Autodesk Inventor part; units mm, degrees
note: some values were not read from the file. Chosen so that the rebuilt part matches the saved one: direction of "Hole2".
(part 7 of 20)
  line L1382 (-10069.986148, -10024.709041) -> (-10070.005021, -10024.908148)
  line L1383 (-10070.235032, -10024.68545) -> (-10069.986148, -10024.709041)
  line L1384 (-10070.235026, -10024.68555) -> (-10070.235032, -10024.68545)
  line L1385 (-10069.009483, -10025.002511) -> (-10070.005021, -10024.908148)
  line L1386 (-10070.235032, -10024.68545) -> (-10070.055742, -10022.793928)
  line L1387 (-10068.562436, -10022.935473) -> (-10068.741726, -10024.826995)
  line L1388 (-10069.787985, -10022.618411) -> (-10068.792448, -10022.712774)
  line L1389 (-10068.562436, -10022.935473) -> (-10068.81132, -10022.911882)
  line L1390 (-10068.81132, -10022.911882) -> (-10068.792448, -10022.712774)
  line L1391 (-10068.792448, -10022.712774) -> (-10068.792441, -10022.712875)
  line L1392 (-10068.56243, -10022.935573) -> (-10068.562436, -10022.935473)
  line L1393 (-10069.787985, -10022.618411) -> (-10069.806858, -10022.817519)
  line L1394 (-10069.806858, -10022.817519) -> (-10070.055742, -10022.793928)
  line L1395 (-10069.967275, -10024.509933) -> (-10069.825731, -10023.016626)
  line L1396 (-10069.825731, -10023.016626) -> (-10068.830193, -10023.11099)
  line L1397 (-10068.830193, -10023.11099) -> (-10068.971738, -10024.604296)
  line L1398 (-10068.971738, -10024.604296) -> (-10069.967275, -10024.509933)
  line L1399 (-10069.666825, -10023.208877) -> (-10069.775092, -10024.351103)
  line L1400 (-10069.825731, -10023.016626) -> (-10069.666825, -10023.208877)
  line L1401 (-10069.967275, -10024.509933) -> (-10069.775092, -10024.351103)
  line L1402 (-10069.775092, -10024.351103) -> (-10069.130635, -10024.412189)
  line L1403 (-10068.971738, -10024.604296) -> (-10069.130635, -10024.412189)
  line L1404 (-10069.130635, -10024.412189) -> (-10069.022367, -10023.269963)
  line L1405 (-10068.830193, -10023.11099) -> (-10069.022367, -10023.269963)
  line L1406 (-10069.022367, -10023.269963) -> (-10069.666825, -10023.208877)
  circle A29 centre (-10069.423446, -10024.071258) radius 0.1
  line L1407 (-10069.258836, -10023.924227) -> (-10069.289393, -10024.246605)
  line L1408 (-10069.289393, -10024.246605) -> (-10069.588054, -10024.218296)
  line L1409 (-10069.289392, -10024.246619) -> (-10069.588054, -10024.21831)
  line L1410 (-10069.588054, -10024.218296) -> (-10069.557498, -10023.895918)
  line L1411 (-10069.557498, -10023.895918) -> (-10069.258836, -10023.924227)
  line L1412 (-10080.829661, -10022.531991) -> (-10080.630553, -10022.531991)
  line L1413 (-10080.630553, -10022.531991) -> (-10080.630553, -10022.781991)
  line L1414 (-10080.630553, -10021.531991) -> (-10080.829661, -10021.531991)
  line L1415 (-10080.630553, -10021.281991) -> (-10080.630553, -10021.531991)
  line L1416 (-10080.829661, -10022.531991) -> (-10080.829661, -10021.531991)
  line L1417 (-10080.630553, -10021.281991) -> (-10078.824469, -10021.281991)
  line L1418 (-10078.824469, -10022.781991) -> (-10080.630553, -10022.781991)
  line L1419 (-10080.431445, -10021.531991) -> (-10079.023383, -10021.531991)
  line L1420 (-10079.023383, -10022.531991) -> (-10080.431445, -10022.531991)
  line L1421 (-10080.431445, -10022.531991) -> (-10080.431445, -10021.531991)
  line L1422 (-10079.680879, -10021.708318) -> (-10080.161579, -10021.708318)
  line L1423 (-10080.431445, -10021.531991) -> (-10080.161579, -10021.708318)
  line L1424 (-10080.161579, -10021.708318) -> (-10080.161579, -10022.355664)
  line L1425 (-10080.431445, -10022.531991) -> (-10080.161579, -10022.355664)
  line L1426 (-10080.161579, -10022.355664) -> (-10079.680879, -10022.355664)
  ellipse E657 centre (-10079.874789, -10022.031991) end of major axis (-10079.874789, -10021.931991) minor radius 0.099554
  ellipse E658 centre (-10079.870072, -10022.031991) end of major axis (-10079.870072, -10021.931991) minor radius 0.099554 (-10079.870072, -10022.131991) -> (-10079.870072, -10021.931991) ccw
  line L1427 (-10079.870072, -10022.131991) -> (-10079.874789, -10022.131991)
  line L1428 (-10079.870072, -10021.931991) -> (-10079.874789, -10021.931991)
  line L1429 (-10079.708883, -10022.181991) -> (-10080.031262, -10022.181991)
  line L1430 (-10079.690018, -10022.181991) -> (-10079.708883, -10022.181991)
  line L1431 (-10080.031262, -10022.181991) -> (-10080.031262, -10021.881991)
  line L1432 (-10080.031262, -10021.881991) -> (-10079.708883, -10021.881991)
  line L1433 (-10079.690018, -10021.881991) -> (-10079.708883, -10021.881991)
  line L1434 (-10079.708883, -10021.881991) -> (-10079.708883, -10022.181991)
  line L1435 (-10079.690018, -10021.881991) -> (-10079.690018, -10022.181991)
  line L1436 (-10070.252033, -10020.246991) -> (-10070.252033, -10020.046991)
  line L1437 (-10070.221551, -10020.246991) -> (-10070.252033, -10020.246991)
  line L1438 (-10070.003148, -10020.046991) -> (-10069.973178, -10020.046991)
  line L1439 (-10070.252033, -10020.046991) -> (-10070.003148, -10020.046991)
  line L1440 (-10071.247575, -10020.046991) -> (-10071.247575, -10020.246991)
  line L1441 (-10071.49646, -10020.046991) -> (-10071.247575, -10020.046991)
  line L1442 (-10070.252033, -10020.246991) -> (-10071.247575, -10020.246991)
  line L1443 (-10071.49646, -10020.046991) -> (-10071.49646, -10018.146991)
  line L1444 (-10070.003148, -10018.146991) -> (-10070.003148, -10020.046991)
  line L1445 (-10071.247575, -10017.946991) -> (-10070.252033, -10017.946991)
  line L1446 (-10070.003148, -10018.146991) -> (-10070.252033, -10018.146991)
  line L1447 (-10070.252033, -10018.146991) -> (-10070.252033, -10017.946991)
  line L1448 (-10070.252033, -10017.946991) -> (-10070.221551, -10017.946991)
  line L1449 (-10069.973178, -10018.146991) -> (-10070.003148, -10018.146991)
  line L1450 (-10071.247575, -10017.946991) -> (-10071.247575, -10018.146991)
  line L1451 (-10071.247575, -10018.146991) -> (-10071.49646, -10018.146991)
  line L1452 (-10071.247575, -10019.846991) -> (-10071.247575, -10018.346991)
  line L1453 (-10071.247575, -10018.346991) -> (-10070.252033, -10018.346991)
  line L1454 (-10070.252033, -10018.346991) -> (-10070.252033, -10019.846991)
  line L1455 (-10070.252033, -10019.846991) -> (-10071.247575, -10019.846991)
  line L1456 (-10071.247575, -10018.346991) -> (-10071.154859, -10018.40757)
  line L1457 (-10071.247575, -10019.846991) -> (-10071.154859, -10019.786412)
  line L1458 (-10070.252033, -10019.846991) -> (-10070.27838, -10019.78979)
  line L1459 (-10070.252033, -10018.346991) -> (-10070.27838, -10018.404192)
  line L1460 (-10068.792448, -10015.481207) -> (-10068.81132, -10015.2821)
  line L1461 (-10068.792441, -10015.481107) -> (-10068.792448, -10015.481207)
  line L1462 (-10068.562436, -10015.258509) -> (-10068.56243, -10015.258409)
  line L1463 (-10068.81132, -10015.2821) -> (-10068.562436, -10015.258509)
  line L1464 (-10069.806858, -10015.376463) -> (-10069.787985, -10015.57557)
  line L1465 (-10070.055742, -10015.400054) -> (-10069.806858, -10015.376463)
  line L1466 (-10068.792448, -10015.481207) -> (-10069.787985, -10015.57557)
  line L1467 (-10070.055742, -10015.400054) -> (-10070.235032, -10013.508532)
  line L1468 (-10068.741726, -10013.366987) -> (-10068.562436, -10015.258509)
  line L1469 (-10070.005021, -10013.285833) -> (-10069.009483, -10013.19147)
  line L1470 (-10070.235032, -10013.508532) -> (-10070.235026, -10013.508431)
  line L1471 (-10070.005021, -10013.285833) -> (-10069.986148, -10013.484941)
  line L1472 (-10069.986148, -10013.484941) -> (-10070.235032, -10013.508532)
  line L1473 (-10070.005014, -10013.285733) -> (-10070.005021, -10013.285833)
  line L1474 (-10068.741726, -10013.366987) -> (-10068.99061, -10013.390578)
  line L1475 (-10068.99061, -10013.390578) -> (-10069.009483, -10013.19147)
  line L1476 (-10069.009483, -10013.19147) -> (-10069.009477, -10013.19137)
  line L1477 (-10068.99061, -10013.390578) -> (-10068.990604, -10013.390478)
  line L1478 (-10068.74172, -10013.366887) -> (-10068.741726, -10013.366987)
  line L1479 (-10069.825731, -10015.177355) -> (-10069.967275, -10013.684048)
  line L1480 (-10069.967275, -10013.684048) -> (-10068.971738, -10013.589685)
  line L1481 (-10068.971738, -10013.589685) -> (-10068.830193, -10015.082992)
  line L1482 (-10068.830193, -10015.082992) -> (-10069.825731, -10015.177355)
  line L1483 (-10069.775092, -10013.842878) -> (-10069.666825, -10014.985105)
  line L1484 (-10069.967275, -10013.684048) -> (-10069.775092, -10013.842878)
  line L1485 (-10069.825731, -10015.177355) -> (-10069.666825, -10014.985105)
  line L1486 (-10069.666825, -10014.985105) -> (-10069.022367, -10014.924019)
  line L1487 (-10068.830193, -10015.082992) -> (-10069.022367, -10014.924019)
  line L1488 (-10069.022367, -10014.924019) -> (-10069.130635, -10013.781793)
  line L1489 (-10068.971738, -10013.589685) -> (-10069.130635, -10013.781793)
  line L1490 (-10069.130635, -10013.781793) -> (-10069.775092, -10013.842878)
  circle A30 centre (-10069.374016, -10014.644209) radius 0.1
  line L1491 (-10069.239964, -10014.468862) -> (-10069.209407, -10014.79124)
  line L1492 (-10069.209407, -10014.79124) -> (-10069.508068, -10014.819549)
  line L1493 (-10069.508068, -10014.819549) -> (-10069.538625, -10014.497171)
  line L1494 (-10069.538625, -10014.497171) -> (-10069.239964, -10014.468862)
  line L1495 (-10069.538624, -10014.497157) -> (-10069.239963, -10014.468848)
  line L1496 (-10051.002001, -10021.596991) -> (-10051.202001, -10021.596991)
  line L1497 (-10051.202001, -10021.596991) -> (-10051.202001, -10021.346991)
  line L1498 (-10051.202001, -10022.596991) -> (-10051.002001, -10022.596991)
  line L1499 (-10051.202001, -10022.846991) -> (-10051.202001, -10022.596991)
  line L1500 (-10051.002001, -10021.596991) -> (-10051.002001, -10022.596991)
  line L1501 (-10051.202001, -10022.846991) -> (-10053.102001, -10022.846991)
  line L1502 (-10053.102001, -10021.346991) -> (-10051.202001, -10021.346991)
  line L1503 (-10053.302001, -10022.596991) -> (-10053.302001, -10021.596991)
  line L1504 (-10053.102001, -10021.346991) -> (-10053.102001, -10021.596991)
  line L1505 (-10053.102001, -10021.596991) -> (-10053.302001, -10021.596991)
  line L1506 (-10053.302001, -10022.596991) -> (-10053.102001, -10022.596991)
  line L1507 (-10053.102001, -10022.596991) -> (-10053.102001, -10022.846991)
  line L1508 (-10051.402001, -10022.596991) -> (-10052.902001, -10022.596991)
  line L1509 (-10052.902001, -10022.596991) -> (-10052.902001, -10021.596991)
  line L1510 (-10052.902001, -10021.596991) -> (-10051.402001, -10021.596991)
  line L1511 (-10051.402001, -10021.596991) -> (-10051.402001, -10022.596991)
  line L1512 (-10052.725674, -10022.420664) -> (-10051.578328, -10022.420664)
  line L1513 (-10052.902001, -10022.596991) -> (-10052.725674, -10022.420664)
  line L1514 (-10051.402001, -10022.596991) -> (-10051.578328, -10022.420664)
  line L1515 (-10051.578328, -10022.420664) -> (-10051.578328, -10021.773318)
  line L1516 (-10051.402001, -10021.596991) -> (-10051.578328, -10021.773318)
  line L1517 (-10051.578328, -10021.773318) -> (-10052.725674, -10021.773318)
  line L1518 (-10052.902001, -10021.596991) -> (-10052.725674, -10021.773318)
  line L1519 (-10052.725674, -10021.773318) -> (-10052.725674, -10022.420664)
  circle A31 centre (-10051.890089, -10022.096991) radius 0.1
  line L1520 (-10052.052001, -10021.946991) -> (-10051.728178, -10021.946991)
  line L1521 (-10051.728178, -10021.946991) -> (-10051.728178, -10022.246991)
  line L1522 (-10051.728178, -10022.246991) -> (-10052.052001, -10022.246991)
  line L1523 (-10052.052001, -10022.246991) -> (-10052.052001, -10021.946991)
  line L1524 (-10061.600001, -10017.946991) -> (-10061.600001, -10018.146991)
  line L1525 (-10061.600001, -10018.146991) -> (-10061.850001, -10018.146991)
  line L1526 (-10060.600001, -10018.146991) -> (-10060.600001, -10017.946991)
  line L1527 (-10060.350001, -10018.146991) -> (-10060.600001, -10018.146991)
  line L1528 (-10061.600001, -10017.946991) -> (-10060.600001, -10017.946991)
  line L1529 (-10060.350001, -10018.146991) -> (-10060.350001, -10020.046991)
  line L1530 (-10061.850001, -10020.046991) -> (-10061.850001, -10018.146991)
  line L1531 (-10060.600001, -10020.246991) -> (-10061.600001, -10020.246991)
  line L1532 (-10061.850001, -10020.046991) -> (-10061.600001, -10020.046991)
  line L1533 (-10061.600001, -10020.046991) -> (-10061.600001, -10020.246991)
  line L1534 (-10060.600001, -10020.246991) -> (-10060.600001, -10020.046991)
  line L1535 (-10060.600001, -10020.046991) -> (-10060.350001, -10020.046991)
  line L1536 (-10060.600001, -10018.346991) -> (-10060.600001, -10019.846991)
  line L1537 (-10060.600001, -10019.846991) -> (-10061.600001, -10019.846991)
  line L1538 (-10061.600001, -10019.846991) -> (-10061.600001, -10018.346991)
  line L1539 (-10061.600001, -10018.346991) -> (-10060.600001, -10018.346991)
  line L1540 (-10060.776328, -10019.670664) -> (-10060.776328, -10018.523318)
  line L1541 (-10060.600001, -10019.846991) -> (-10060.776328, -10019.670664)
  line L1542 (-10060.600001, -10018.346991) -> (-10060.776328, -10018.523318)
  line L1543 (-10060.776328, -10018.523318) -> (-10061.423674, -10018.523318)
  line L1544 (-10061.600001, -10018.346991) -> (-10061.423674, -10018.523318)
  line L1545 (-10061.423674, -10018.523318) -> (-10061.423674, -10019.670664)
  line L1546 (-10061.600001, -10019.846991) -> (-10061.423674, -10019.670664)
  line L1547 (-10061.423674, -10019.670664) -> (-10060.776328, -10019.670664)
  circle A32 centre (-10061.100001, -10018.835079) radius 0.1
  line L1548 (-10061.250001, -10018.996991) -> (-10061.250001, -10018.673168)
  line L1549 (-10061.250001, -10018.673168) -> (-10060.950001, -10018.673168)
  line L1550 (-10060.950001, -10018.673168) -> (-10060.950001, -10018.996991)
  line L1551 (-10060.950001, -10018.996991) -> (-10061.250001, -10018.996991)
  line L1552 (-10051.002001, -10015.596991) -> (-10051.202001, -10015.596991)
  line L1553 (-10051.202001, -10015.596991) -> (-10051.202001, -10015.346991)
  line L1554 (-10051.202001, -10016.596991) -> (-10051.002001, -10016.596991)
  line L1555 (-10051.202001, -10016.846991) -> (-10051.202001, -10016.596991)
  line L1556 (-10051.002001, -10015.596991) -> (-10051.002001, -10016.596991)
  line L1557 (-10051.202001, -10016.846991) -> (-10053.102001, -10016.846991)
  line L1558 (-10053.102001, -10015.346991) -> (-10051.202001, -10015.346991)
  line L1559 (-10053.302001, -10016.596991) -> (-10053.302001, -10015.596991)
  line L1560 (-10053.102001, -10015.346991) -> (-10053.102001, -10015.596991)
  line L1561 (-10053.102001, -10015.596991) -> (-10053.302001, -10015.596991)
  line L1562 (-10053.302001, -10016.596991) -> (-10053.102001, -10016.596991)
  line L1563 (-10053.102001, -10016.596991) -> (-10053.102001, -10016.846991)
  line L1564 (-10051.402001, -10016.596991) -> (-10052.902001, -10016.596991)
  line L1565 (-10052.902001, -10016.596991) -> (-10052.902001, -10015.596991)
  line L1566 (-10052.902001, -10015.596991) -> (-10051.402001, -10015.596991)
  line L1567 (-10051.402001, -10015.596991) -> (-10051.402001, -10016.596991)
  line L1568 (-10052.725674, -10016.420664) -> (-10051.578328, -10016.420664)
  line L1569 (-10052.902001, -10016.596991) -> (-10052.725674, -10016.420664)
  line L1570 (-10051.402001, -10016.596991) -> (-10051.578328, -10016.420664)
  line L1571 (-10051.578328, -10016.420664) -> (-10051.578328, -10015.773318)
  line L1572 (-10051.402001, -10015.596991) -> (-10051.578328, -10015.773318)
  line L1573 (-10051.578328, -10015.773318) -> (-10052.725674, -10015.773318)
  line L1574 (-10052.902001, -10015.596991) -> (-10052.725674, -10015.773318)
  line L1575 (-10052.725674, -10015.773318) -> (-10052.725674, -10016.420664)
  circle A33 centre (-10051.890089, -10016.096991) radius 0.1
  line L1576 (-10052.052001, -10015.946991) -> (-10051.728178, -10015.946991)
  line L1577 (-10051.728178, -10015.946991) -> (-10051.728178, -10016.246991)
  line L1578 (-10051.728178, -10016.246991) -> (-10052.052001, -10016.246991)
  line L1579 (-10052.052001, -10016.246991) -> (-10052.052001, -10015.946991)
  line L1580 (-10079.023383, -10015.661991) -> (-10078.824469, -10015.661991)
  line L1581 (-10078.824469, -10015.661991) -> (-10078.824469, -10015.411991)
  line L1582 (-10078.824469, -10016.661991) -> (-10079.023383, -10016.661991)
  line L1583 (-10078.824469, -10016.911991) -> (-10078.824469, -10016.661991)
  line L1584 (-10079.023383, -10015.661991) -> (-10079.023383, -10016.661991)
  line L1585 (-10078.824469, -10016.911991) -> (-10077.066524, -10016.911991)
  line L1586 (-10077.066524, -10015.411991) -> (-10078.824469, -10015.411991)
  line L1587 (-10078.625555, -10016.661991) -> (-10077.265175, -10016.661991)
  line L1588 (-10078.625555, -10015.661991) -> (-10078.625555, -10016.661991)
  line L1589 (-10077.265175, -10015.661991) -> (-10078.625555, -10015.661991)
  line L1590 (-10078.625555, -10016.661991) -> (-10078.372051, -10016.50203)
  line L1591 (-10078.625555, -10015.661991) -> (-10078.372051, -10015.821952)
  ellipse E659 centre (-10078.062063, -10016.161991) end of major axis (-10078.062063, -10016.261991) minor radius 0.099457
  ellipse E660 centre (-10078.056859, -10016.161991) end of major axis (-10078.056859, -10016.261991) minor radius 0.099457 (-10078.056859, -10016.261991) -> (-10078.056859, -10016.061991) ccw
  line L1592 (-10078.062063, -10016.061991) -> (-10078.056859, -10016.061991)
  line L1593 (-10078.062063, -10016.261991) -> (-10078.056859, -10016.261991)
  line L1594 (-10077.895827, -10016.011991) -> (-10078.217892, -10016.011991)
  line L1595 (-10077.88528, -10016.011991) -> (-10077.895827, -10016.011991)
  line L1596 (-10078.217892, -10016.011991) -> (-10078.217892, -10016.311991)
  line L1597 (-10078.217892, -10016.311991) -> (-10077.895827, -10016.311991)
  line L1598 (-10077.88528, -10016.311991) -> (-10077.895827, -10016.311991)
  line L1599 (-10077.895827, -10016.311991) -> (-10077.895827, -10016.011991)
  line L1600 (-10077.691531, -10011.315342) -> (-10077.890346, -10011.336143)
  line L1601 (-10077.890346, -10011.336143) -> (-10077.890422, -10011.336371)
  line L1602 (-10077.890422, -10011.336371) -> (-10077.691508, -10011.31556)
  line L1603 (-10077.691508, -10011.31556) -> (-10077.717522, -10011.066917)
  line L1604 (-10077.717522, -10011.066917) -> (-10077.717446, -10011.066689)
  line L1605 (-10077.58745, -10012.310131) -> (-10077.786364, -10012.330942)
  line L1606 (-10077.561436, -10012.558774) -> (-10077.58745, -10012.310131)
  line L1607 (-10075.973217, -10010.884197) -> (-10077.717446, -10011.066689)
  line L1608 (-10075.498774, -10012.091381) -> (-10075.526412, -10011.827228)
  line L1609 (-10077.890422, -10011.336371) -> (-10077.786364, -10012.330942)
  line L1610 (-10077.561436, -10012.558774) -> (-10075.67175, -10012.361064)
  line L1611 (-10075.49885, -10012.09161) -> (-10075.602908, -10011.097038)
  line L1612 (-10075.827837, -10010.869207) -> (-10077.717522, -10011.066917)
  line L1613 (-10075.671674, -10012.360836) -> (-10075.697666, -10012.112411)
  line L1614 (-10075.67175, -10012.361064) -> (-10075.671674, -10012.360836)
  line L1615 (-10075.697765, -10012.112421) -> (-10075.67175, -10012.361064)
  line L1616 (-10075.49885, -10012.09161) -> (-10075.697765, -10012.112421)
  line L1617 (-10075.498774, -10012.091381) -> (-10075.49885, -10012.09161)
  line L1618 (-10075.801822, -10011.11785) -> (-10075.602908, -10011.097038)
  line L1619 (-10075.827837, -10010.869207) -> (-10075.801822, -10011.11785)
  line L1620 (-10077.388536, -10012.289319) -> (-10075.896679, -10012.133233)
  line L1621 (-10077.492594, -10011.294748) -> (-10077.388536, -10012.289319)
  line L1622 (-10076.000737, -10011.138661) -> (-10077.492594, -10011.294748)
  line L1623 (-10075.896679, -10012.133233) -> (-10076.000737, -10011.138661)
  line L1624 (-10076.090343, -10011.976048) -> (-10077.23146, -10012.095439)
  line L1625 (-10077.388536, -10012.289319) -> (-10077.23146, -10012.095439)
  line L1626 (-10075.896679, -10012.133233) -> (-10076.090343, -10011.976048)
  line L1627 (-10077.23146, -10012.095439) -> (-10077.298821, -10011.451607)
  line L1628 (-10077.492594, -10011.294748) -> (-10077.298821, -10011.451607)
  line L1629 (-10077.298821, -10011.451607) -> (-10076.157704, -10011.332216)
  line L1630 (-10076.000737, -10011.138661) -> (-10076.157704, -10011.332216)
  line L1631 (-10076.157704, -10011.332216) -> (-10076.090343, -10011.976048)
  circle A34 centre (-10076.955085, -10011.741122) radius 0.1
  line L1632 (-10076.809659, -10011.57508) -> (-10077.131723, -10011.608776)
  line L1633 (-10076.809648, -10011.575048) -> (-10076.809659, -10011.57508)
  line L1634 (-10076.809648, -10011.575048) -> (-10077.131713, -10011.608744)
  line L1635 (-10077.131713, -10011.608744) -> (-10077.131723, -10011.608776)
  line L1636 (-10077.131723, -10011.608776) -> (-10077.100506, -10011.907148)
  line L1637 (-10077.100506, -10011.907148) -> (-10076.778441, -10011.873452)
  line L1638 (-10076.77843, -10011.873419) -> (-10076.778441, -10011.873452)
  line L1639 (-10076.778441, -10011.873452) -> (-10076.809659, -10011.57508)
  line L1640 (-10076.77843, -10011.873419) -> (-10076.809648, -10011.575048)
  line L1641 (-10077.265175, -10015.661991) -> (-10077.066524, -10015.661991)
  line L1642 (-10077.066524, -10015.661991) -> (-10077.066524, -10015.411991)
  line L1643 (-10077.066524, -10016.661991) -> (-10077.265175, -10016.661991)
  line L1644 (-10077.066524, -10016.911991) -> (-10077.066524, -10016.661991)
  line L1645 (-10075.017046, -10015.661991) -> (-10075.017046, -10015.411991)
  line L1646 (-10075.179332, -10015.661991) -> (-10074.98068, -10015.661991)
  line L1647 (-10075.179332, -10015.411991) -> (-10075.179332, -10015.661991)
  line L1648 (-10074.98068, -10015.661991) -> (-10074.818395, -10015.661991)
  line L1649 (-10075.017046, -10015.411991) -> (-10075.179332, -10015.411991)
  line L1650 (-10074.818395, -10016.661991) -> (-10074.818395, -10015.661991)
  line L1651 (-10077.265175, -10015.661991) -> (-10077.265175, -10016.661991)
  line L1652 (-10077.066524, -10016.911991) -> (-10075.179332, -10016.911991)
  line L1653 (-10074.98068, -10016.661991) -> (-10074.98068, -10015.661991)
  line L1654 (-10075.179332, -10015.411991) -> (-10077.066524, -10015.411991)
  line L1655 (-10075.017046, -10016.911991) -> (-10075.017046, -10016.661991)
  line L1656 (-10075.179332, -10016.911991) -> (-10075.017046, -10016.911991)
  line L1657 (-10075.179332, -10016.661991) -> (-10075.179332, -10016.911991)
  line L1658 (-10074.98068, -10016.661991) -> (-10075.179332, -10016.661991)
  line L1659 (-10074.818395, -10016.661991) -> (-10074.98068, -10016.661991)
  line L1660 (-10076.867872, -10016.661991) -> (-10075.377984, -10016.661991)
  line L1661 (-10076.867872, -10015.661991) -> (-10076.867872, -10016.661991)
  line L1662 (-10075.377984, -10015.661991) -> (-10076.867872, -10015.661991)
  line L1663 (-10075.377984, -10016.661991) -> (-10075.377984, -10015.661991)
  line L1664 (-10075.437204, -10016.485664) -> (-10076.576815, -10016.485664)
  line L1665 (-10076.867872, -10016.661991) -> (-10076.576815, -10016.485664)
  line L1666 (-10075.377984, -10016.661991) -> (-10075.437204, -10016.485664)
  line L1667 (-10076.576815, -10016.485664) -> (-10076.576815, -10015.838318)
  line L1668 (-10076.867872, -10015.661991) -> (-10076.576815, -10015.838318)
  line L1669 (-10076.576815, -10015.838318) -> (-10075.437204, -10015.838318)
  line L1670 (-10075.377984, -10015.661991) -> (-10075.437204, -10015.838318)
  line L1671 (-10075.437204, -10015.838318) -> (-10075.437204, -10016.485664)
  ellipse E661 centre (-10076.296135, -10016.161991) end of major axis (-10076.296135, -10016.261991) minor radius 0.099326
  ellipse E662 centre (-10076.290339, -10016.161991) end of major axis (-10076.290339, -10016.261991) minor radius 0.099326 (-10076.290339, -10016.261991) -> (-10076.290339, -10016.061991) ccw
  line L1672 (-10076.296135, -10016.061991) -> (-10076.290339, -10016.061991)
  line L1673 (-10076.296135, -10016.261991) -> (-10076.290339, -10016.261991)
  line L1674 (-10076.129519, -10016.011991) -> (-10076.451159, -10016.011991)
  line L1675 (-10076.106335, -10016.011991) -> (-10076.129519, -10016.011991)
  line L1676 (-10076.451159, -10016.011991) -> (-10076.451159, -10016.311991)
  line L1677 (-10076.451159, -10016.311991) -> (-10076.129519, -10016.311991)
  line L1678 (-10076.106335, -10016.311991) -> (-10076.129519, -10016.311991)
  line L1679 (-10076.129519, -10016.311991) -> (-10076.129519, -10016.011991)
  line L1680 (-10076.106335, -10016.311991) -> (-10076.106335, -10016.011991)
  line L1681 (-10076.003508, -10010.624332) -> (-10076.003562, -10010.624474)
  line L1682 (-10076.003562, -10010.624474) -> (-10075.804914, -10010.601264)
  line L1683 (-10075.804914, -10010.601264) -> (-10075.833925, -10010.352953)
  line L1684 (-10075.833925, -10010.352953) -> (-10075.833871, -10010.352812)
  line L1685 (-10073.946708, -10010.132322) -> (-10075.833871, -10010.352812)
  line L1686 (-10073.715814, -10010.385094) -> (-10073.719047, -10010.357424)
  line L1687 (-10076.003562, -10010.624474) -> (-10075.973192, -10010.884415)
  line L1688 (-10075.52651, -10011.827239) -> (-10073.772692, -10011.622329)
  line L1689 (-10073.603055, -10011.350809) -> (-10073.719102, -10010.357565)
  line L1690 (-10073.946762, -10010.132464) -> (-10075.833925, -10010.352953)
  line L1691 (-10073.920953, -10010.352758) -> (-10073.946708, -10010.132322)
  line L1692 (-10073.719047, -10010.357424) -> (-10073.815719, -10010.368718)
  line L1693 (-10073.917751, -10010.380775) -> (-10073.719102, -10010.357565)
  line L1694 (-10073.946762, -10010.132464) -> (-10073.917751, -10010.380775)
  line L1695 (-10073.917751, -10010.380775) -> (-10073.917696, -10010.380633)
  line L1696 (-10073.719102, -10010.357565) -> (-10073.719047, -10010.357424)
  line L1697 (-10073.946708, -10010.132322) -> (-10073.946762, -10010.132464)
  line L1698 (-10073.772692, -10011.622329) -> (-10073.772637, -10011.622188)
  line L1699 (-10073.801703, -10011.374018) -> (-10073.772692, -10011.622329)
  line L1700 (-10073.603055, -10011.350809) -> (-10073.801703, -10011.374018)
  line L1701 (-10073.603, -10011.350667) -> (-10073.603055, -10011.350809)
  line L1702 (-10075.490218, -10011.571299) -> (-10074.000352, -10011.397228)
  line L1703 (-10075.606265, -10010.578055) -> (-10075.490218, -10011.571299)
  line L1704 (-10074.116399, -10010.403984) -> (-10075.606265, -10010.578055)
  line L1705 (-10074.000352, -10011.397228) -> (-10074.116399, -10010.403984)
  line L1706 (-10074.195911, -10011.242453) -> (-10075.335505, -10011.375599)
  line L1707 (-10075.490218, -10011.571299) -> (-10075.335505, -10011.375599)
  line L1708 (-10074.000352, -10011.397228) -> (-10074.195911, -10011.242453)
  line L1709 (-10075.335505, -10011.375599) -> (-10075.410628, -10010.732627)
  line L1710 (-10075.606265, -10010.578055) -> (-10075.410628, -10010.732627)
  line L1711 (-10075.410628, -10010.732627) -> (-10074.271034, -10010.599481)
  line L1712 (-10074.116399, -10010.403984) -> (-10074.271034, -10010.599481)
  line L1713 (-10074.271034, -10010.599481) -> (-10074.195911, -10011.242453)
  circle A35 centre (-10075.063421, -10011.017959) radius 0.1
  line L1714 (-10074.920009, -10010.850179) -> (-10075.241644, -10010.887757)
  line L1715 (-10074.920001, -10010.850158) -> (-10074.920009, -10010.850179)
  line L1716 (-10074.920001, -10010.850158) -> (-10075.241636, -10010.887737)
  line L1717 (-10075.241636, -10010.887737) -> (-10075.241644, -10010.887757)
  line L1718 (-10075.241644, -10010.887757) -> (-10075.20683, -10011.18573)
  line L1719 (-10075.20683, -10011.18573) -> (-10074.885195, -10011.148152)
  line L1720 (-10074.885187, -10011.148131) -> (-10074.885195, -10011.148152)
  line L1721 (-10074.885195, -10011.148152) -> (-10074.920009, -10010.850179)
  line L1722 (-10074.885187, -10011.148131) -> (-10074.920001, -10010.850158)
  line L1723 (-10080.829661, -10015.661991) -> (-10080.630553, -10015.661991)
  line L1724 (-10080.630553, -10015.661991) -> (-10080.630553, -10015.411991)
  line L1725 (-10080.630553, -10016.661991) -> (-10080.829661, -10016.661991)
  line L1726 (-10080.630553, -10016.911991) -> (-10080.630553, -10016.661991)
  line L1727 (-10080.829661, -10015.661991) -> (-10080.829661, -10016.661991)
  line L1728 (-10080.630553, -10016.911991) -> (-10078.824469, -10016.911991)
  line L1729 (-10078.824469, -10015.411991) -> (-10080.630553, -10015.411991)
  line L1730 (-10080.431445, -10016.661991) -> (-10079.023383, -10016.661991)
  line L1731 (-10080.431445, -10015.661991) -> (-10080.431445, -10016.661991)
  line L1732 (-10079.023383, -10015.661991) -> (-10080.431445, -10015.661991)
  line L1733 (-10079.680879, -10016.485664) -> (-10080.161579, -10016.485664)
  line L1734 (-10080.431445, -10016.661991) -> (-10080.161579, -10016.485664)
  line L1735 (-10080.161579, -10016.485664) -> (-10080.161579, -10015.838318)
  line L1736 (-10080.431445, -10015.661991) -> (-10080.161579, -10015.838318)
  line L1737 (-10080.161579, -10015.838318) -> (-10079.680879, -10015.838318)
  ellipse E663 centre (-10079.874789, -10016.161991) end of major axis (-10079.874789, -10016.261991) minor radius 0.099554
  ellipse E664 centre (-10079.870072, -10016.161991) end of major axis (-10079.870072, -10016.261991) minor radius 0.099554 (-10079.870072, -10016.261991) -> (-10079.870072, -10016.061991) ccw
  line L1738 (-10079.874789, -10016.061991) -> (-10079.870072, -10016.061991)
  line L1739 (-10079.874789, -10016.261991) -> (-10079.870072, -10016.261991)
  line L1740 (-10079.708883, -10016.011991) -> (-10080.031262, -10016.011991)
  line L1741 (-10079.690018, -10016.011991) -> (-10079.708883, -10016.011991)
  line L1742 (-10080.031262, -10016.011991) -> (-10080.031262, -10016.311991)
  line L1743 (-10080.031262, -10016.311991) -> (-10079.708883, -10016.311991)
  line L1744 (-10079.690018, -10016.311991) -> (-10079.708883, -10016.311991)
  line L1745 (-10079.708883, -10016.311991) -> (-10079.708883, -10016.011991)
  line L1746 (-10079.690018, -10016.311991) -> (-10079.690018, -10016.011991)
  line L1747 (-10079.603594, -10011.900303) -> (-10079.802686, -10011.919175)
  line L1748 (-10079.802686, -10011.919175) -> (-10079.802692, -10011.919275)
  line L1749 (-10079.802692, -10011.919275) -> (-10079.603585, -10011.900402)
  line L1750 (-10079.603585, -10011.900402) -> (-10079.627175, -10011.651518)
  line L1751 (-10079.627175, -10011.651518) -> (-10079.627169, -10011.651417)
  line L1752 (-10079.509221, -10012.89594) -> (-10079.708329, -10012.914813)
  line L1753 (-10079.485631, -10013.144825) -> (-10079.509221, -10012.89594)
  line L1754 (-10079.407047, -10011.630553) -> (-10079.627169, -10011.651417)
  line L1755 (-10079.802692, -10011.919275) -> (-10079.708329, -10012.914813)
  line L1756 (-10079.485631, -10013.144825) -> (-10077.594109, -10012.965534)
  line L1757 (-10077.418592, -10012.697777) -> (-10077.433041, -10012.54534)
  line L1758 (-10077.874828, -10011.48542) -> (-10079.627175, -10011.651518)
  line L1759 (-10077.594109, -10012.965534) -> (-10077.594103, -10012.965434)
  line L1760 (-10077.6177, -10012.71665) -> (-10077.594109, -10012.965534)
  line L1761 (-10077.418592, -10012.697777) -> (-10077.6177, -10012.71665)
  line L1762 (-10077.418586, -10012.697677) -> (-10077.418592, -10012.697777)
  line L1763 (-10079.310114, -10012.877067) -> (-10077.816807, -10012.735523)
  line L1764 (-10079.404477, -10011.88153) -> (-10079.310114, -10012.877067)
  line L1765 (-10077.91117, -10011.739985) -> (-10079.404477, -10011.88153)
  line L1766 (-10077.816807, -10012.735523) -> (-10077.91117, -10011.739985)
  line L1767 (-10078.008982, -10012.57655) -> (-10079.151208, -10012.684817)
  line L1768 (-10079.310114, -10012.877067) -> (-10079.151208, -10012.684817)
  line L1769 (-10077.816807, -10012.735523) -> (-10078.008982, -10012.57655)
  line L1770 (-10079.151208, -10012.684817) -> (-10079.212294, -10012.040359)
  line L1771 (-10079.404477, -10011.88153) -> (-10079.212294, -10012.040359)
  line L1772 (-10079.212294, -10012.040359) -> (-10078.070067, -10011.932092)
  line L1773 (-10077.91117, -10011.739985) -> (-10078.070067, -10011.932092)
  line L1774 (-10078.070067, -10011.932092) -> (-10078.008982, -10012.57655)
  circle A36 centre (-10078.871381, -10012.333187) radius 0.1
  line L1775 (-10078.724347, -10012.168574) -> (-10079.046725, -10012.199131)
  line L1776 (-10078.724346, -10012.16856) -> (-10079.046724, -10012.199117)
  line L1777 (-10079.046725, -10012.199131) -> (-10079.018416, -10012.497793)
  line L1778 (-10079.018416, -10012.497793) -> (-10078.696038, -10012.467236)
  line L1779 (-10078.696038, -10012.467236) -> (-10078.724347, -10012.168574)
  ellipse E665 centre (-10075.730106, -10029.62245) end of major axis (-10075.669515, -10030.82092) minor radius 0.214474 (-10075.933672, -10028.865824) -> (-10075.631613, -10030.799013) ccw
  ellipse E666 centre (-10075.533577, -10029.612514) end of major axis (-10075.483085, -10030.611239) minor radius 0.178729 (-10075.711061, -10029.080492) -> (-10075.384751, -10030.398789) ccw
  line L1780 (-10075.4515, -10030.592983) -> (-10075.631613, -10030.799013)
  ellipse E667 centre (-10075.533577, -10029.612514) end of major axis (-10075.495708, -10030.361558) minor radius 0.134046 (-10075.671866, -10029.337058) -> (-10075.41406, -10030.151964) ccw
  line L1781 (-10075.669515, -10030.82092) -> (-10076.518016, -10030.863817)
  ellipse E668 centre (-10075.730106, -10008.571531) end of major axis (-10075.669515, -10007.373062) minor radius 0.214474 (-10075.631613, -10007.394969) -> (-10075.933672, -10009.328157) ccw
  ellipse E669 centre (-10075.533577, -10008.581467) end of major axis (-10075.483085, -10007.582743) minor radius 0.178729 (-10075.384751, -10007.795193) -> (-10075.711061, -10009.11349) ccw
  line L1782 (-10075.4515, -10007.600998) -> (-10075.631613, -10007.394969)
  ellipse E670 centre (-10075.533577, -10008.581467) end of major axis (-10075.495708, -10007.832424) minor radius 0.134046 (-10075.41406, -10008.042018) -> (-10075.671866, -10008.856924) ccw
  line L1783 (-10075.669515, -10007.373062) -> (-10076.518016, -10007.330164)
  ellipse E671 centre (-10090.417065, -10019.096991) end of major axis (-10090.417065, -10019.663411) minor radius 0.563895 (-10089.989225, -10018.728017) -> (-10089.989225, -10019.465964) ccw
  line L1784 (-10090.80989, -10019.210594) -> (-10090.711422, -10018.812073)
  line L1785 (-10090.711422, -10018.812073) -> (-10090.318598, -10018.69847)
  line L1786 (-10090.318598, -10018.69847) -> (-10090.048204, -10018.960194)
  line L1787 (-10090.080668, -10019.211762) -> (-10090.122709, -10019.381909)
  line L1788 (-10090.122709, -10019.381909) -> (-10090.515533, -10019.495512)
  line L1789 (-10090.515533, -10019.495512) -> (-10090.80989, -10019.210594)
  line L1790 (-10090.711422, -10018.812073) -> (-10090.621727, -10018.812073)
  line L1791 (-10090.720635, -10019.210594) -> (-10090.80989, -10019.210594)
  spline S53 degree 3 poles (-10045.596901, -10030.692025) (-10045.596275, -10030.687279) (-10045.594915, -10030.676953) (-10045.585272, -10030.662297) (-10045.570743, -10030.647725) (-10045.550423, -10030.633362) (-10045.524771, -10030.619481) (-10045.482006, -10030.600847) (-10045.432986, -10030.585045) (-10045.378486, -10030.571429) (-10045.314115, -10030.55807) (-10045.225805, -10030.544735) (-10045.114584, -10030.535371) (-10045.000001, -10030.532033) (-10044.885417, -10030.535371) (-10044.774196, -10030.544735) (-10044.685886, -10030.55807) (-10044.621515, -10030.571429) (-10044.567015, -10030.585045) (-10044.517995, -10030.600847) (-10044.475231, -10030.619481) (-10044.449578, -10030.633362) (-10044.429258, -10030.647725) (-10044.41473, -10030.662297) (-10044.405087, -10030.676953) (-10044.403726, -10030.687279) (-10044.403101, -10030.692025) knots 0 0 0 0 0.01106677 0.02407754 0.03992786 0.05913986 0.0819337 0.10802006 0.16805875 0.20201508 0.23929564 0.3216678 0.41056278 0.5 0.58943722 0.6783322 0.76070436 0.79798492 0.83194125 0.89197994 0.9180663 0.94086014 0.96007214 0.97592246 0.98893323 1 1 1 1
  spline S54 degree 3 poles (-10044.403101, -10030.692025) (-10044.40371, -10030.696687) (-10044.40502, -10030.706704) (-10044.4147, -10030.72062) (-10044.429303, -10030.733859) (-10044.449659, -10030.74639) (-10044.475326, -10030.758015) (-10044.518218, -10030.77314) (-10044.567213, -10030.785232) (-10044.621593, -10030.795282) (-10044.686052, -10030.804929) (-10044.774405, -10030.814185) (-10044.885516, -10030.820497) (-10045.000001, -10030.822685) (-10045.114485, -10030.820497) (-10045.225596, -10030.814185) (-10045.313949, -10030.804929) (-10045.378409, -10030.795282) (-10045.432789, -10030.785232) (-10045.481783, -10030.77314) (-10045.524676, -10030.758015) (-10045.550342, -10030.74639) (-10045.570698, -10030.733859) (-10045.585301, -10030.72062) (-10045.594981, -10030.706704) (-10045.596291, -10030.696687) (-10045.596901, -10030.692025) knots 0 0 0 0 0.01099744 0.02362844 0.03895388 0.0576141 0.07990846 0.10559498 0.1652091 0.19914929 0.2365432 0.31951534 0.40940333 0.5 0.59059667 0.68048466 0.7634568 0.80085071 0.8347909 0.89440502 0.92009154 0.9423859 0.96104612 0.97637156 0.98900256 1 1 1 1
  spline S55 degree 3 poles (-10044.403101, -10007.501957) (-10044.403726, -10007.506703) (-10044.405087, -10007.517028) (-10044.41473, -10007.531684) (-10044.429258, -10007.546257) (-10044.449578, -10007.56062) (-10044.475231, -10007.574501) (-10044.517995, -10007.593135) (-10044.567015, -10007.608936) (-10044.621515, -10007.622553) (-10044.685886, -10007.635912) (-10044.774196, -10007.649246) (-10044.885417, -10007.65861) (-10045.000001, -10007.661949) (-10045.114584, -10007.65861) (-10045.225805, -10007.649246) (-10045.314115, -10007.635912) (-10045.378486, -10007.622553) (-10045.432986, -10007.608936) (-10045.482006, -10007.593135) (-10045.524771, -10007.574501) (-10045.550423, -10007.56062) (-10045.570743, -10007.546257) (-10045.585272, -10007.531684) (-10045.594915, -10007.517028) (-10045.596275, -10007.506703) (-10045.596901, -10007.501957) knots 0 0 0 0 0.01106677 0.02407754 0.03992786 0.05913986 0.0819337 0.10802006 0.16805875 0.20201508 0.23929564 0.3216678 0.41056278 0.5 0.58943722 0.6783322 0.76070436 0.79798492 0.83194125 0.89197994 0.9180663 0.94086014 0.96007214 0.97592246 0.98893323 1 1 1 1
  spline S56 degree 3 poles (-10045.596901, -10007.501957) (-10045.596291, -10007.497295) (-10045.594981, -10007.487278) (-10045.585301, -10007.473362) (-10045.570698, -10007.460123) (-10045.550342, -10007.447592) (-10045.524676, -10007.435966) (-10045.481783, -10007.420841) (-10045.432789, -10007.40875) (-10045.378409, -10007.3987) (-10045.313949, -10007.389053) (-10045.225596, -10007.379797) (-10045.114485, -10007.373484) (-10045.000001, -10007.371296) (-10044.885516, -10007.373484) (-10044.774405, -10007.379797) (-10044.686052, -10007.389053) (-10044.621593, -10007.3987) (-10044.567213, -10007.40875) (-10044.518218, -10007.420841) (-10044.475326, -10007.435966) (-10044.449659, -10007.447592) (-10044.429303, -10007.460123) (-10044.4147, -10007.473362) (-10044.40502, -10007.487278) (-10044.40371, -10007.497295) (-10044.403101, -10007.501957) knots 0 0 0 0 0.01099744 0.02362844 0.03895388 0.0576141 0.07990846 0.10559498 0.1652091 0.19914929 0.2365432 0.31951534 0.40940333 0.5 0.59059667 0.68048466 0.7634568 0.80085071 0.8347909 0.89440502 0.92009154 0.9423859 0.96104612 0.97637156 0.98900256 1 1 1 1
  line L1792 (-10042.592001, -10023.310235) -> (-10042.500001, -10023.310235)
  line L1793 (-10042.500001, -10028.251222) -> (-10043.100001, -10028.251222)
  line L1794 (-10042.500001, -10023.310235) -> (-10042.500001, -10028.251222)
  line L1795 (-10042.500001, -10014.883746) -> (-10042.592001, -10014.883746)
  line L1796 (-10042.500001, -10009.94276) -> (-10042.500001, -10014.883746)
  line L1797 (-10043.100001, -10009.94276) -> (-10042.500001, -10009.94276)
  line L1798 (-10043.100001, -10023.096991) -> (-10043.100001, -10028.251222)
  line L1799 (-10043.100001, -10009.94276) -> (-10043.100001, -10015.096991)
  line L1800 (-10042.500001, -10007.146991) -> (-10042.500001, -10009.94276)
  line L1801 (-10042.500001, -10028.251222) -> (-10042.500001, -10031.046991)
  line L1802 (-10047.500001, -10015.096991) -> (-10047.500001, -10007.146991)
  line L1803 (-10047.500001, -10031.046991) -> (-10047.500001, -10023.096991)
  line L1804 (-10042.500001, -10031.046991) -> (-10047.500001, -10031.046991)
  line L1805 (-10042.500001, -10007.146991) -> (-10047.500001, -10007.146991)
  line L1806 (-10042.500001, -10014.883746) -> (-10042.500001, -10015.193606)
  line L1807 (-10042.500001, -10015.193606) -> (-10042.592001, -10015.193606)
  line L1808 (-10042.500001, -10015.193606) -> (-10042.500001, -10023.310235)
  line L1809 (-10057.500001, -10028.179355) -> (-10057.500001, -10022.422127)
  line L1810 (-10057.500001, -10015.771854) -> (-10057.500001, -10010.014627)
  line L1811 (-10057.500001, -10008.446758) -> (-10057.500001, -10007.883695)
  line L1812 (-10057.500001, -10030.310287) -> (-10057.500001, -10029.747223)
  line L1813 (-10047.500001, -10007.883695) -> (-10057.500001, -10007.883695)
  line L1814 (-10057.500001, -10030.310287) -> (-10047.500001, -10030.310287)
  spline S57 degree 3 poles (-10050.100962, -10027.864783) (-10050.211197, -10027.864524) (-10050.435123, -10027.861121) (-10050.767559, -10027.84302) (-10051.040759, -10027.812873) (-10051.230079, -10027.779538) (-10051.322295, -10027.745051) (-10051.384762, -10027.721643) (-10051.38723, -10027.672416) (-10051.347186, -10027.644814) (-10051.266604, -10027.609981) (-10051.080384, -10027.572853) (-10050.807061, -10027.541371) (-10050.47559, -10027.523435) (-10050.142265, -10027.519039) (-10049.809344, -10027.526598) (-10049.475461, -10027.546591) (-10049.203421, -10027.578487) (-10049.013747, -10027.614292) (-10048.922488, -10027.646705) (-10048.856797, -10027.670533) (-10048.856597, -10027.719885) (-10048.898082, -10027.746237) (-10048.97872, -10027.777012) (-10049.164478, -10027.814102) (-10049.436909, -10027.843332) (-10049.769074, -10027.86089) (-10049.991679, -10027.86504) (-10050.100962, -10027.864783) knots 0 0 0 0 0.06370705 0.12949472 0.19191208 0.22368799 0.2382902 0.25135028 0.25660425 0.26301775 0.27714857 0.30853838 0.37103998 0.43687849 0.50002298 0.56369496 0.62938323 0.69283553 0.72316052 0.73857311 0.75180992 0.75696152 0.7632602 0.77795176 0.80804313 0.87131401 0.93684349 1 1 1 1
  spline S58 degree 3 poles (-10050.182554, -10030.060957) (-10050.405273, -10030.060342) (-10050.729126, -10030.049978) (-10051.125529, -10030.049938) (-10051.283629, -10030.012187) (-10051.377423, -10030.021414) (-10051.387465, -10029.984778) (-10051.307021, -10029.97405) (-10051.219699, -10029.95551) (-10050.999402, -10029.940474) (-10050.729582, -10029.927005) (-10050.395734, -10029.91968) (-10049.949321, -10029.915609) (-10049.516441, -10029.931275) (-10049.119331, -10029.934805) (-10048.960444, -10029.974512) (-10048.865885, -10029.965204) (-10048.855387, -10030.002544) (-10048.937825, -10030.011165) (-10049.024857, -10030.029173) (-10049.245962, -10030.041401) (-10049.623295, -10030.057463) (-10049.959576, -10030.061572) (-10050.182554, -10030.060957) knots 0 0 0 0 0.13139199 0.19506211 0.22486648 0.236537 0.23877104 0.24363774 0.27264718 0.30298792 0.36807806 0.43503205 0.49911295 0.63103815 0.69471519 0.72474683 0.73665002 0.73889428 0.74387281 0.77307947 0.80345172 0.86845517 1 1 1 1
  spline S59 degree 3 poles (-10050.182554, -10010.673065) (-10050.292885, -10010.67274) (-10050.517502, -10010.669684) (-10050.846374, -10010.647846) (-10051.127031, -10010.618394) (-10051.293616, -10010.570971) (-10051.385476, -10010.534878) (-10051.386744, -10010.485874) (-10051.324598, -10010.442539) (-10051.213572, -10010.412045) (-10051.001395, -10010.375226) (-10050.725282, -10010.348038) (-10050.393956, -10010.331632) (-10050.060673, -10010.327435) (-10049.727295, -10010.334454) (-10049.3981, -10010.354007) (-10049.118556, -10010.384551) (-10048.950953, -10010.428292) (-10048.859058, -10010.460524) (-10048.855333, -10010.510005) (-10048.920879, -10010.553678) (-10049.029979, -10010.581415) (-10049.242379, -10010.622784) (-10049.517313, -10010.649949) (-10049.850482, -10010.669029) (-10050.073336, -10010.673387) (-10050.182554, -10010.673065) knots 0 0 0 0 0.06377364 0.12947571 0.19191728 0.22251596 0.23572674 0.24098241 0.24712107 0.27642984 0.3084167 0.37100213 0.43691035 0.50001881 0.5637377 0.62924964 0.69193924 0.72212339 0.73538665 0.74053978 0.7469427 0.77702751 0.80721947 0.87118814 0.93686953 1 1 1 1
  line L1815 (-10057.500001, -10010.014627) -> (-10057.500001, -10008.446758)
  line L1816 (-10057.500001, -10029.747223) -> (-10057.500001, -10028.179355)
  spline S60 degree 3 poles (-10050.100962, -10008.275766) (-10050.324865, -10008.275074) (-10050.6589, -10008.273158) (-10051.037887, -10008.248807) (-10051.230877, -10008.240154) (-10051.316184, -10008.216565) (-10051.38198, -10008.223094) (-10051.385322, -10008.185715) (-10051.339999, -10008.182295) (-10051.267717, -10008.162825) (-10051.075982, -10008.154028) (-10050.807338, -10008.139516) (-10050.475013, -10008.133991) (-10050.029532, -10008.132162) (-10049.583837, -10008.135588) (-10049.206937, -10008.156617) (-10049.012203, -10008.164021) (-10048.929848, -10008.185594) (-10048.858207, -10008.178062) (-10048.859063, -10008.215696) (-10048.904648, -10008.218799) (-10048.977552, -10008.238306) (-10049.168367, -10008.249836) (-10049.544367, -10008.272462) (-10049.878451, -10008.276453) (-10050.100962, -10008.275766) knots 0 0 0 0 0.13209168 0.19547472 0.22735918 0.24158397 0.25296859 0.25518606 0.26025608 0.27356013 0.30485536 0.36824052 0.43535326 0.4998067 0.63172546 0.69607433 0.72644443 0.74148548 0.75299654 0.75519516 0.76033444 0.77439415 0.80449955 0.86873005 1 1 1 1
  line L1817 (-10055.030001, -10015.096991) -> (-10062.350001, -10017.096991)
  line L1818 (-10062.350001, -10021.096991) -> (-10055.030001, -10023.096991)
  line L1819 (-10043.608001, -10015.096991) -> (-10055.030001, -10015.096991)
  line L1820 (-10043.608001, -10023.096991) -> (-10055.030001, -10023.096991)
  line L1821 (-10062.350001, -10017.096991) -> (-10062.350001, -10021.096991)
  line L1822 (-10043.608001, -10015.096991) -> (-10042.592001, -10015.096991)
  line L1823 (-10043.608001, -10023.096991) -> (-10042.592001, -10023.096991)
  line L1824 (-10042.592001, -10015.096991) -> (-10042.592001, -10023.096991)
  line L1825 (-10042.592001, -10027.221959) -> (-10042.592001, -10027.396819)
  line L1826 (-10043.100001, -10027.221959) -> (-10042.592001, -10027.221959)
  line L1827 (-10042.592001, -10023.519552) -> (-10042.592001, -10027.221959)
  line L1828 (-10042.592001, -10023.519552) -> (-10042.592001, -10023.096991)
  line L1829 (-10042.592001, -10015.096991) -> (-10042.592001, -10014.67443)
  line L1830 (-10042.592001, -10010.972023) -> (-10042.592001, -10014.67443)
  line L1831 (-10043.100001, -10010.972023) -> (-10042.592001, -10010.972023)
  line L1832 (-10042.592001, -10010.797163) -> (-10042.592001, -10010.972023)
  line L1833 (-10043.100001, -10027.396819) -> (-10042.592001, -10027.396819)
  line L1834 (-10043.100001, -10010.797163) -> (-10042.592001, -10010.797163)
  line L1835 (-10039.500001, -10030.096991) -> (-10039.500001, -10008.096991)
  line L1836 (-10006.500001, -10030.096991) -> (-10006.500001, -10008.096991)
  line L1837 (-10006.500001, -10030.096991) -> (-10039.500001, -10030.096991)
  line L1838 (-10006.500001, -10008.096991) -> (-10039.500001, -10008.096991)
  line L1839 (-10039.500001, -10028.495476) -> (-10042.500001, -10028.495476)
  line L1840 (-10039.500001, -10026.395476) -> (-10042.500001, -10026.395476)
  line L1841 (-10039.500001, -10020.146991) -> (-10042.500001, -10020.146991)
  line L1842 (-10039.500001, -10018.046991) -> (-10042.500001, -10018.046991)
  line L1843 (-10039.500001, -10011.798506) -> (-10042.500001, -10011.798506)
  line L1844 (-10039.500001, -10009.698506) -> (-10042.500001, -10009.698506)
  point P0 (-10071.573564, -10018.382119)
  point P1 (-10089.414469, -10025.238171)
  point P2 (-10089.470693, -10025.105442)
  point P3 (-10089.524117, -10024.974692)
  point P4 (-10089.574789, -10024.84581)
  point P5 (-10089.668048, -10024.593222)
  point P6 (-10089.710002, -10026.541042)
  point P7 (-10089.707897, -10026.58022)
  point P8 (-10089.706792, -10026.618096)
  point P9 (-10089.706736, -10026.654459)
  point P10 (-10089.707778, -10026.689103)
  point P11 (-10089.709929, -10026.721877)
  point P12 (-10089.713143, -10026.75273)
  point P13 (-10089.717369, -10026.781619)
  point P14 (-10089.722554, -10026.808502)
  point P15 (-10089.728647, -10026.833334)
  point P16 (-10089.735597, -10026.856075)
  point P17 (-10089.74335, -10026.87668)
  point P18 (-10089.751883, -10026.895163)
  point P19 (-10089.761396, -10026.91201)
  point P20 (-10089.771919, -10026.927303)
  point P21 (-10089.56433, -10022.118968)
  point P22 (-10089.633681, -10021.99281)
  point P23 (-10089.700058, -10021.868329)
  point P24 (-10089.76352, -10021.74542)
  point P25 (-10089.88191, -10021.503906)
  point P26 (-10089.88191, -10016.690075)
  point P27 (-10089.76352, -10016.448562)
  point P28 (-10089.700058, -10016.325653)
  point P29 (-10089.633681, -10016.201172)
  point P30 (-10089.56433, -10016.075014)
  point P31 (-10089.668048, -10013.60076)
  point P32 (-10089.574789, -10013.348171)
  point P33 (-10089.524117, -10013.219289)
  point P34 (-10089.470693, -10013.08854)
  point P35 (-10089.414469, -10012.955811)
  point P36 (-10089.771901, -10011.267674)
  point P37 (-10089.761101, -10011.283731)
  point P38 (-10089.751232, -10011.301595)
  point P39 (-10089.742311, -10011.321249)
  point P40 (-10089.734354, -10011.342676)